Autodesk Fusion 360 part; units mm, degrees
(part 3 of 5)
  spline S32 degree 5 poles (96.0186, 106.2511) (96.0621, 106.2993) (96.1478, 106.3966) (96.2726, 106.5457) (96.4317, 106.7503) (96.6205, 107.0141) (96.8023, 107.2836) (96.9796, 107.5565) (97.1546, 107.8314) (97.328, 108.1075) (97.4996, 108.3849) (97.6689, 108.664) (97.8352, 108.9454) (97.9978, 109.2294) (98.1569, 109.5161) (98.3127, 109.8051) (98.4657, 110.0962) (98.6162, 110.389) (98.7647, 110.6831) (98.9112, 110.9786) (99.0558, 111.2754) (99.1982, 111.5737) (99.3383, 111.8734) (99.4762, 112.1746) (99.6118, 112.4773) (99.7453, 112.7815) (99.8767, 113.0869) (100.0061, 113.3936) (100.1336, 113.7015) (100.2592, 114.0106) (100.383, 114.3207) (100.5049, 114.6321) (100.6249, 114.9445) (100.7431, 115.2581) (100.8594, 115.5727) (100.974, 115.8885) (101.0867, 116.2052) (101.1977, 116.523) (101.3069, 116.8418) (101.4144, 117.1615) (101.5203, 117.4822) (101.6244, 117.8038) (101.7269, 118.1263) (101.8276, 118.4498) (101.9268, 118.7742) (102.0242, 119.0994) (102.1201, 119.4255) (102.2143, 119.7524) (102.307, 120.0802) (102.398, 120.4088) (102.4875, 120.7382) (102.5754, 121.0684) (102.6617, 121.3994) (102.7465, 121.7312) (102.8297, 122.0637) (102.9114, 122.397) (102.9916, 122.731) (103.0703, 123.0657) (103.1474, 123.4011) (103.2231, 123.7373) (103.2972, 124.0741) (103.3699, 124.4117) (103.4411, 124.7499) (103.5108, 125.0888) (103.5791, 125.4283) (103.6459, 125.7685) (103.7112, 126.1093) (103.7751, 126.4508) (103.8376, 126.7928) (103.8986, 127.1355) (103.9582, 127.4788) (104.0048, 127.7539) (104.039, 127.9605) (104.0616, 128.0984) (104.0728, 128.1673) knots 0 0 0 0 0 0 0.01428571 0.02857143 0.04285714 0.05714286 0.07142857 0.08571429 0.1 0.11428571 0.12857143 0.14285714 0.15714286 0.17142857 0.18571429 0.2 0.21428571 0.22857143 0.24285714 0.25714286 0.27142857 0.28571429 0.3 0.31428571 0.32857143 0.34285714 0.35714286 0.37142857 0.38571429 0.4 0.41428571 0.42857143 0.44285714 0.45714286 0.47142857 0.48571429 0.5 0.51428571 0.52857143 0.54285714 0.55714286 0.57142857 0.58571429 0.6 0.61428571 0.62857143 0.64285714 0.65714286 0.67142857 0.68571429 0.7 0.71428571 0.72857143 0.74285714 0.75714286 0.77142857 0.78571429 0.8 0.81428571 0.82857143 0.84285714 0.85714286 0.87142857 0.88571429 0.9 0.91428571 0.92857143 0.94285714 0.95714286 0.97142857 0.98571429 1 1 1 1 1 1
  arc A66 (104.0728, 128.1673) -> (96.8641, 133.6987) centre (0, 0) ccw
  spline S33 degree 5 poles (96.8641, 133.6987) (96.8004, 133.6701) (96.6731, 133.6126) (96.4824, 133.526) (96.2287, 133.4099) (95.9125, 133.2634) (95.5973, 133.1158) (95.2831, 132.9669) (94.9698, 132.8168) (94.6575, 132.6655) (94.3462, 132.5129) (94.0359, 132.3591) (93.7266, 132.2041) (93.4184, 132.0478) (93.1111, 131.8902) (92.805, 131.7314) (92.4998, 131.5713) (92.1958, 131.41) (91.8928, 131.2474) (91.5909, 131.0835) (91.2902, 130.9183) (90.9905, 130.7518) (90.692, 130.5841) (90.3946, 130.415) (90.0984, 130.2447) (89.8034, 130.073) (89.5096, 129.9) (89.2169, 129.7257) (88.9255, 129.55) (88.6354, 129.373) (88.3464, 129.1947) (88.0588, 129.015) (87.7724, 128.8339) (87.4874, 128.6515) (87.2037, 128.4677) (86.9213, 128.2824) (86.6403, 128.0958) (86.3607, 127.9078) (86.0825, 127.7184) (85.8057, 127.5275) (85.5303, 127.3352) (85.2565, 127.1414) (84.9842, 126.9461) (84.7135, 126.7492) (84.4443, 126.5509) (84.1768, 126.3511) (83.9108, 126.1497) (83.6464, 125.9469) (83.3836, 125.7425) (83.1225, 125.5365) (82.8633, 125.3289) (82.606, 125.1196) (82.3507, 124.9084) (82.0975, 124.6954) (81.8463, 124.4807) (81.597, 124.2643) (81.3495, 124.0463) (81.1038, 123.8267) (80.86, 123.6055) (80.6184, 123.3824) (80.3795, 123.1571) (80.1438, 122.9293) (79.9116, 122.6986) (79.6828, 122.4652) (79.457, 122.2295) (79.2335, 121.9919) (79.0117, 121.7529) (78.7915, 121.5128) (78.5737, 121.2708) (78.3604, 121.0256) (78.1545, 120.7749) (77.998, 120.5683) (77.8863, 120.4091) (77.8145, 120.3011) (77.7792, 120.2466) knots -1 -1 -1 -1 -1 -1 -0.98571429 -0.97142857 -0.95714286 -0.94285714 -0.92857143 -0.91428571 -0.9 -0.88571429 -0.87142857 -0.85714286 -0.84285714 -0.82857143 -0.81428571 -0.8 -0.78571429 -0.77142857 -0.75714286 -0.74285714 -0.72857143 -0.71428571 -0.7 -0.68571429 -0.67142857 -0.65714286 -0.64285714 -0.62857143 -0.61428571 -0.6 -0.58571429 -0.57142857 -0.55714286 -0.54285714 -0.52857143 -0.51428571 -0.5 -0.48571429 -0.47142857 -0.45714286 -0.44285714 -0.42857143 -0.41428571 -0.4 -0.38571429 -0.37142857 -0.35714286 -0.34285714 -0.32857143 -0.31428571 -0.3 -0.28571429 -0.27142857 -0.25714286 -0.24285714 -0.22857143 -0.21428571 -0.2 -0.18571429 -0.17142857 -0.15714286 -0.14285714 -0.12857143 -0.11428571 -0.1 -0.08571429 -0.07142857 -0.05714286 -0.04285714 -0.02857143 -0.01428571 0 0 0 0 0 0
  line L33 (77.7792, 120.2466) -> (75.8689, 117.2932)
  arc A67 (73.1275, 116.6848) -> (75.8689, 117.2932) centre (74.1896, 118.3795) ccw
  arc A68 (73.1275, 116.6848) -> (64.4882, 121.6727) centre (0, 0) ccw
  arc A69 (63.6445, 124.351) -> (64.4882, 121.6727) centre (65.4248, 123.4398) ccw
  line L34 (63.6445, 124.351) -> (65.247, 127.4821)
  spline S34 degree 5 poles (65.247, 127.4821) (65.2766, 127.5399) (65.3342, 127.6561) (65.4162, 127.8324) (65.5168, 128.0712) (65.631, 128.3749) (65.7368, 128.6822) (65.8374, 128.9918) (65.9353, 129.3026) (66.0313, 129.6142) (66.1253, 129.9265) (66.2166, 130.2399) (66.3044, 130.5548) (66.388, 130.8712) (66.4674, 131.1893) (66.5431, 131.5088) (66.6155, 131.8296) (66.6852, 132.1513) (66.7525, 132.4739) (66.8175, 132.7972) (66.8803, 133.1213) (66.9407, 133.4463) (66.9985, 133.772) (67.0537, 134.0987) (67.1064, 134.4262) (67.1565, 134.7545) (67.2044, 135.0836) (67.25, 135.4133) (67.2935, 135.7437) (67.3349, 136.0747) (67.3741, 136.4064) (67.4113, 136.7386) (67.4464, 137.0715) (67.4794, 137.405) (67.5103, 137.739) (67.5392, 138.0736) (67.5661, 138.4088) (67.5911, 138.7445) (67.6141, 139.0806) (67.6352, 139.4173) (67.6544, 139.7544) (67.6718, 140.0921) (67.6872, 140.4301) (67.7009, 140.7687) (67.7127, 141.1076) (67.7227, 141.447) (67.7309, 141.7868) (67.7373, 142.127) (67.7419, 142.4676) (67.7448, 142.8085) (67.746, 143.1499) (67.7454, 143.4916) (67.7431, 143.8336) (67.7392, 144.176) (67.7335, 144.5188) (67.7262, 144.8618) (67.7171, 145.2052) (67.7065, 145.5489) (67.6942, 145.8929) (67.6803, 146.2371) (67.6647, 146.5817) (67.6475, 146.9266) (67.6288, 147.2717) (67.6084, 147.6171) (67.5865, 147.9627) (67.5629, 148.3086) (67.5378, 148.6547) (67.5112, 149.001) (67.483, 149.3476) (67.4533, 149.6944) (67.422, 150.0414) (67.3957, 150.3192) (67.3754, 150.5276) (67.3615, 150.6666) (67.3545, 150.7362) knots 0 0 0 0 0 0 0.01428571 0.02857143 0.04285714 0.05714286 0.07142857 0.08571429 0.1 0.11428571 0.12857143 0.14285714 0.15714286 0.17142857 0.18571429 0.2 0.21428571 0.22857143 0.24285714 0.25714286 0.27142857 0.28571429 0.3 0.31428571 0.32857143 0.34285714 0.35714286 0.37142857 0.38571429 0.4 0.41428571 0.42857143 0.44285714 0.45714286 0.47142857 0.48571429 0.5 0.51428571 0.52857143 0.54285714 0.55714286 0.57142857 0.58571429 0.6 0.61428571 0.62857143 0.64285714 0.65714286 0.67142857 0.68571429 0.7 0.71428571 0.72857143 0.74285714 0.75714286 0.77142857 0.78571429 0.8 0.81428571 0.82857143 0.84285714 0.85714286 0.87142857 0.88571429 0.9 0.91428571 0.92857143 0.94285714 0.95714286 0.97142857 0.98571429 1 1 1 1 1 1
  arc A70 (67.3545, 150.7362) -> (58.9598, 154.2133) centre (0, 0) ccw
  spline S35 degree 5 poles (58.9598, 154.2133) (58.9056, 154.1692) (58.7975, 154.0807) (58.6357, 153.9477) (58.4208, 153.7698) (58.1533, 153.5466) (57.887, 153.3224) (57.622, 153.0973) (57.3583, 152.8712) (57.0958, 152.6442) (56.8346, 152.4163) (56.5747, 152.1874) (56.316, 151.9576) (56.0587, 151.7268) (55.8028, 151.4951) (55.5481, 151.2625) (55.2948, 151.0289) (55.0429, 150.7943) (54.7923, 150.5588) (54.5432, 150.3224) (54.2954, 150.085) (54.049, 149.8467) (53.8041, 149.6074) (53.5606, 149.3671) (53.3186, 149.1259) (53.0781, 148.8837) (52.839, 148.6405) (52.6015, 148.3964) (52.3655, 148.1513) (52.131, 147.9053) (51.8981, 147.6582) (51.6667, 147.4102) (51.437, 147.1612) (51.2089, 146.9112) (50.9824, 146.6602) (50.7576, 146.4082) (50.5345, 146.1552) (50.313, 145.9012) (50.0933, 145.6463) (49.8754, 145.3902) (49.6592, 145.1332) (49.4448, 144.8751) (49.2324, 144.616) (49.0218, 144.3558) (48.8132, 144.0946) (48.6064, 143.8323) (48.4016, 143.569) (48.1987, 143.3046) (47.9978, 143.0392) (47.799, 142.7727) (47.6023, 142.505) (47.408, 142.2362) (47.216, 141.9662) (47.0265, 141.695) (46.8395, 141.4225) (46.6547, 141.149) (46.472, 140.8743) (46.2915, 140.5987) (46.1133, 140.3219) (45.9377, 140.0439) (45.7653, 139.7644) (45.5965, 139.4833) (45.4319, 139.2004) (45.2713, 138.9158) (45.1143, 138.6296) (44.9599, 138.3422) (44.8074, 138.054) (44.6569, 137.7651) (44.5092, 137.475) (44.3666, 137.1829) (44.2326, 136.8874) (44.135, 136.6474) (44.0682, 136.4648) (44.0268, 136.3418) (44.0069, 136.2801) knots -1 -1 -1 -1 -1 -1 -0.98571429 -0.97142857 -0.95714286 -0.94285714 -0.92857143 -0.91428571 -0.9 -0.88571429 -0.87142857 -0.85714286 -0.84285714 -0.82857143 -0.81428571 -0.8 -0.78571429 -0.77142857 -0.75714286 -0.74285714 -0.72857143 -0.71428571 -0.7 -0.68571429 -0.67142857 -0.65714286 -0.64285714 -0.62857143 -0.61428571 -0.6 -0.58571429 -0.57142857 -0.55714286 -0.54285714 -0.52857143 -0.51428571 -0.5 -0.48571429 -0.47142857 -0.45714286 -0.44285714 -0.42857143 -0.41428571 -0.4 -0.38571429 -0.37142857 -0.35714286 -0.34285714 -0.32857143 -0.31428571 -0.3 -0.28571429 -0.27142857 -0.25714286 -0.24285714 -0.22857143 -0.21428571 -0.2 -0.18571429 -0.17142857 -0.15714286 -0.14285714 -0.12857143 -0.11428571 -0.1 -0.08571429 -0.07142857 -0.05714286 -0.04285714 -0.02857143 -0.01428571 0 0 0 0 0 0
  line L35 (44.0069, 136.2801) -> (42.926, 132.9329)
  arc A71 (40.4355, 131.6356) -> (42.926, 132.9329) centre (41.0228, 133.5475) ccw
  arc A72 (40.4355, 131.6356) -> (30.7996, 134.2176) centre (0, 0) ccw
  arc A73 (29.2914, 136.5863) -> (30.7996, 134.2176) centre (31.247, 136.1669) ccw
  line L36 (29.2914, 136.5863) -> (30.029, 140.0254)
  spline S36 degree 5 poles (30.029, 140.0254) (30.0426, 140.0889) (30.0682, 140.2161) (30.1017, 140.4076) (30.1371, 140.6643) (30.1688, 140.9872) (30.1914, 141.3114) (30.2085, 141.6365) (30.2226, 141.962) (30.2347, 142.2878) (30.2447, 142.6139) (30.2518, 142.9402) (30.255, 143.267) (30.2539, 143.5944) (30.2483, 143.9222) (30.2387, 144.2504) (30.2257, 144.579) (30.2097, 144.9078) (30.1912, 145.2368) (30.1703, 145.5659) (30.1471, 145.8952) (30.1213, 146.2247) (30.0928, 146.5543) (30.0616, 146.8842) (30.0277, 147.2141) (29.9912, 147.5442) (29.9523, 147.8745) (29.911, 148.2048) (29.8675, 148.5352) (29.8217, 148.8657) (29.7739, 149.1962) (29.7238, 149.5267) (29.6715, 149.8573) (29.6171, 150.188) (29.5605, 150.5186) (29.5018, 150.8493) (29.441, 151.18) (29.3782, 151.5107) (29.3135, 151.8414) (29.2467, 152.172) (29.178, 152.5027) (29.1074, 152.8333) (29.0349, 153.1638) (28.9604, 153.4944) (28.8841, 153.8248) (28.8059, 154.1552) (28.7259, 154.4856) (28.644, 154.8158) (28.5603, 155.146) (28.4749, 155.4761) (28.3877, 155.8061) (28.2987, 156.136) (28.208, 156.4658) (28.1155, 156.7955) (28.0213, 157.1251) (27.9254, 157.4546) (27.8279, 157.7839) (27.7286, 158.1132) (27.6277, 158.4422) (27.5252, 158.7712) (27.4209, 159.1) (27.3151, 159.4286) (27.2077, 159.7571) (27.0986, 160.0855) (26.9879, 160.4136) (26.8757, 160.7417) (26.7619, 161.0695) (26.6465, 161.3971) (26.5296, 161.7246) (26.4111, 162.0519) (26.2911, 162.379) (26.1938, 162.6405) (26.1202, 162.8366) (26.0708, 162.9672) (26.046, 163.0326) knots 0 0 0 0 0 0 0.01428571 0.02857143 0.04285714 0.05714286 0.07142857 0.08571429 0.1 0.11428571 0.12857143 0.14285714 0.15714286 0.17142857 0.18571429 0.2 0.21428571 0.22857143 0.24285714 0.25714286 0.27142857 0.28571429 0.3 0.31428571 0.32857143 0.34285714 0.35714286 0.37142857 0.38571429 0.4 0.41428571 0.42857143 0.44285714 0.45714286 0.47142857 0.48571429 0.5 0.51428571 0.52857143 0.54285714 0.55714286 0.57142857 0.58571429 0.6 0.61428571 0.62857143 0.64285714 0.65714286 0.67142857 0.68571429 0.7 0.71428571 0.72857143 0.74285714 0.75714286 0.77142857 0.78571429 0.8 0.81428571 0.82857143 0.84285714 0.85714286 0.87142857 0.88571429 0.9 0.91428571 0.92857143 0.94285714 0.95714286 0.97142857 0.98571429 1 1 1 1 1 1
  arc A74 (26.046, 163.0326) -> (17.0374, 164.2186) centre (0, 0) ccw
  spline S37 degree 5 poles (17.0374, 164.2186) (16.9966, 164.1619) (16.915, 164.0484) (16.7932, 163.8781) (16.6316, 163.6507) (16.431, 163.3658) (16.2318, 163.0803) (16.0341, 162.7943) (15.8379, 162.5077) (15.6431, 162.2205) (15.4498, 161.9327) (15.2579, 161.6443) (15.0676, 161.3554) (14.8788, 161.0659) (14.6915, 160.7758) (14.5057, 160.4852) (14.3215, 160.194) (14.1389, 159.9023) (13.9578, 159.61) (13.7783, 159.3171) (13.6005, 159.0237) (13.4242, 158.7297) (13.2495, 158.4351) (13.0765, 158.1401) (12.9052, 157.8444) (12.7355, 157.5482) (12.5676, 157.2515) (12.4013, 156.9542) (12.2368, 156.6564) (12.0739, 156.358) (11.9129, 156.0591) (11.7536, 155.7597) (11.5962, 155.4597) (11.4406, 155.1592) (11.2868, 154.8581) (11.1349, 154.5565) (10.9848, 154.2544) (10.8367, 153.9518) (10.6904, 153.6486) (10.5461, 153.3449) (10.4039, 153.0407) (10.2636, 152.7359) (10.1254, 152.4306) (9.9894, 152.1248) (9.8555, 151.8185) (9.7237, 151.5116) (9.594, 151.2043) (9.4664, 150.8964) (9.3411, 150.588) (9.218, 150.2791) (9.0973, 149.9697) (8.9791, 149.6597) (8.8636, 149.3492) (8.7508, 149.0382) (8.6406, 148.7266) (8.5329, 148.4145) (8.4276, 148.102) (8.3246, 147.789) (8.224, 147.4755) (8.1264, 147.1615) (8.0321, 146.847) (7.9419, 146.5318) (7.8561, 146.2159) (7.7747, 145.8994) (7.6971, 145.5823) (7.6223, 145.2648) (7.5497, 144.947) (7.479, 144.6289) (7.4114, 144.3105) (7.3493, 143.9914) (7.2964, 143.6714) (7.2641, 143.4142) (7.247, 143.2205) (7.2388, 143.0911) (7.2355, 143.0263) knots -1 -1 -1 -1 -1 -1 -0.98571429 -0.97142857 -0.95714286 -0.94285714 -0.92857143 -0.91428571 -0.9 -0.88571429 -0.87142857 -0.85714286 -0.84285714 -0.82857143 -0.81428571 -0.8 -0.78571429 -0.77142857 -0.75714286 -0.74285714 -0.72857143 -0.71428571 -0.7 -0.68571429 -0.67142857 -0.65714286 -0.64285714 -0.62857143 -0.61428571 -0.6 -0.58571429 -0.57142857 -0.55714286 -0.54285714 -0.52857143 -0.51428571 -0.5 -0.48571429 -0.47142857 -0.45714286 -0.44285714 -0.42857143 -0.41428571 -0.4 -0.38571429 -0.37142857 -0.35714286 -0.34285714 -0.32857143 -0.31428571 -0.3 -0.28571429 -0.27142857 -0.25714286 -0.24285714 -0.22857143 -0.21428571 -0.2 -0.18571429 -0.17142857 -0.15714286 -0.14285714 -0.12857143 -0.11428571 -0.1 -0.08571429 -0.07142857 -0.05714286 -0.04285714 -0.02857143 -0.01428571 0 0 0 0 0 0
  line L37 (7.2355, 143.0263) -> (7.0578, 139.5134)
  arc A75 (4.9879, 137.6157) -> (7.0578, 139.5134) centre (5.0603, 139.6144) ccw
  arc A76 (4.9879, 137.6157) -> (-4.9879, 137.6157) centre (0, 0) ccw
  arc A77 (-7.0578, 139.5134) -> (-4.9879, 137.6157) centre (-5.0603, 139.6144) ccw
  line L38 (-7.0578, 139.5134) -> (-7.2355, 143.0263)
  spline S38 degree 5 poles (-7.2355, 143.0263) (-7.2388, 143.0911) (-7.247, 143.2205) (-7.2641, 143.4142) (-7.2964, 143.6714) (-7.3493, 143.9914) (-7.4114, 144.3105) (-7.479, 144.6289) (-7.5497, 144.947) (-7.6223, 145.2648) (-7.6971, 145.5823) (-7.7747, 145.8994) (-7.8561, 146.2159) (-7.9419, 146.5318) (-8.0321, 146.847) (-8.1264, 147.1615) (-8.224, 147.4755) (-8.3246, 147.789) (-8.4276, 148.102) (-8.5329, 148.4145) (-8.6406, 148.7266) (-8.7508, 149.0382) (-8.8636, 149.3492) (-8.9791, 149.6597) (-9.0973, 149.9697) (-9.218, 150.2791) (-9.3411, 150.588) (-9.4664, 150.8964) (-9.594, 151.2043) (-9.7237, 151.5116) (-9.8555, 151.8185) (-9.9894, 152.1248) (-10.1254, 152.4306) (-10.2636, 152.7359) (-10.4039, 153.0407) (-10.5461, 153.3449) (-10.6904, 153.6486) (-10.8367, 153.9518) (-10.9848, 154.2544) (-11.1349, 154.5565) (-11.2868, 154.8581) (-11.4406, 155.1592) (-11.5962, 155.4597) (-11.7536, 155.7597) (-11.9129, 156.0591) (-12.0739, 156.358) (-12.2368, 156.6564) (-12.4013, 156.9542) (-12.5676, 157.2515) (-12.7355, 157.5482) (-12.9052, 157.8444) (-13.0765, 158.1401) (-13.2495, 158.4351) (-13.4242, 158.7297) (-13.6005, 159.0237) (-13.7783, 159.3171) (-13.9578, 159.61) (-14.1389, 159.9023) (-14.3215, 160.194) (-14.5057, 160.4852) (-14.6915, 160.7758) (-14.8788, 161.0659) (-15.0676, 161.3554) (-15.2579, 161.6443) (-15.4498, 161.9327) (-15.6431, 162.2205) (-15.8379, 162.5077) (-16.0341, 162.7943) (-16.2318, 163.0803) (-16.431, 163.3658) (-16.6316, 163.6507) (-16.7932, 163.8781) (-16.915, 164.0484) (-16.9966, 164.1619) (-17.0374, 164.2186) knots 0 0 0 0 0 0 0.01428571 0.02857143 0.04285714 0.05714286 0.07142857 0.08571429 0.1 0.11428571 0.12857143 0.14285714 0.15714286 0.17142857 0.18571429 0.2 0.21428571 0.22857143 0.24285714 0.25714286 0.27142857 0.28571429 0.3 0.31428571 0.32857143 0.34285714 0.35714286 0.37142857 0.38571429 0.4 0.41428571 0.42857143 0.44285714 0.45714286 0.47142857 0.48571429 0.5 0.51428571 0.52857143 0.54285714 0.55714286 0.57142857 0.58571429 0.6 0.61428571 0.62857143 0.64285714 0.65714286 0.67142857 0.68571429 0.7 0.71428571 0.72857143 0.74285714 0.75714286 0.77142857 0.78571429 0.8 0.81428571 0.82857143 0.84285714 0.85714286 0.87142857 0.88571429 0.9 0.91428571 0.92857143 0.94285714 0.95714286 0.97142857 0.98571429 1 1 1 1 1 1
  arc A78 (-17.0374, 164.2186) -> (-26.046, 163.0326) centre (0, 0) ccw
  spline S39 degree 5 poles (-26.046, 163.0326) (-26.0708, 162.9672) (-26.1202, 162.8366) (-26.1938, 162.6405) (-26.2911, 162.379) (-26.4111, 162.0519) (-26.5296, 161.7246) (-26.6465, 161.3971) (-26.7619, 161.0695) (-26.8757, 160.7417) (-26.9879, 160.4136) (-27.0986, 160.0855) (-27.2077, 159.7571) (-27.3151, 159.4286) (-27.4209, 159.1) (-27.5252, 158.7712) (-27.6277, 158.4422) (-27.7286, 158.1132) (-27.8279, 157.7839) (-27.9254, 157.4546) (-28.0213, 157.1251) (-28.1155, 156.7955) (-28.208, 156.4658) (-28.2987, 156.136) (-28.3877, 155.8061) (-28.4749, 155.4761) (-28.5603, 155.146) (-28.644, 154.8158) (-28.7259, 154.4856) (-28.8059, 154.1552) (-28.8841, 153.8248) (-28.9604, 153.4944) (-29.0349, 153.1638) (-29.1074, 152.8333) (-29.178, 152.5027) (-29.2467, 152.172) (-29.3135, 151.8414) (-29.3782, 151.5107) (-29.441, 151.18) (-29.5018, 150.8493) (-29.5605, 150.5186) (-29.6171, 150.188) (-29.6715, 149.8573) (-29.7238, 149.5267) (-29.7739, 149.1962) (-29.8217, 148.8657) (-29.8675, 148.5352) (-29.911, 148.2048) (-29.9523, 147.8745) (-29.9912, 147.5442) (-30.0277, 147.2141) (-30.0616, 146.8842) (-30.0928, 146.5543) (-30.1213, 146.2247) (-30.1471, 145.8952) (-30.1703, 145.5659) (-30.1912, 145.2368) (-30.2097, 144.9078) (-30.2257, 144.579) (-30.2387, 144.2504) (-30.2483, 143.9222) (-30.2539, 143.5944) (-30.255, 143.267) (-30.2518, 142.9402) (-30.2447, 142.6139) (-30.2347, 142.2878) (-30.2226, 141.962) (-30.2085, 141.6365) (-30.1914, 141.3114) (-30.1688, 140.9872) (-30.1371, 140.6643) (-30.1017, 140.4076) (-30.0682, 140.2161) (-30.0426, 140.0889) (-30.029, 140.0254) knots -1 -1 -1 -1 -1 -1 -0.98571429 -0.97142857 -0.95714286 -0.94285714 -0.92857143 -0.91428571 -0.9 -0.88571429 -0.87142857 -0.85714286 -0.84285714 -0.82857143 -0.81428571 -0.8 -0.78571429 -0.77142857 -0.75714286 -0.74285714 -0.72857143 -0.71428571 -0.7 -0.68571429 -0.67142857 -0.65714286 -0.64285714 -0.62857143 -0.61428571 -0.6 -0.58571429 -0.57142857 -0.55714286 -0.54285714 -0.52857143 -0.51428571 -0.5 -0.48571429 -0.47142857 -0.45714286 -0.44285714 -0.42857143 -0.41428571 -0.4 -0.38571429 -0.37142857 -0.35714286 -0.34285714 -0.32857143 -0.31428571 -0.3 -0.28571429 -0.27142857 -0.25714286 -0.24285714 -0.22857143 -0.21428571 -0.2 -0.18571429 -0.17142857 -0.15714286 -0.14285714 -0.12857143 -0.11428571 -0.1 -0.08571429 -0.07142857 -0.05714286 -0.04285714 -0.02857143 -0.01428571 0 0 0 0 0 0
  line L39 (-30.029, 140.0254) -> (-29.2914, 136.5863)
  arc A79 (-30.7996, 134.2176) -> (-29.2914, 136.5863) centre (-31.247, 136.1669) ccw
  arc A80 (-30.7996, 134.2176) -> (-40.4355, 131.6356) centre (0, 0) ccw
  arc A81 (-42.926, 132.9329) -> (-40.4355, 131.6356) centre (-41.0228, 133.5475) ccw
  line L40 (-42.926, 132.9329) -> (-44.0069, 136.2801)
  spline S40 degree 5 poles (-44.0069, 136.2801) (-44.0268, 136.3418) (-44.0682, 136.4648) (-44.135, 136.6474) (-44.2326, 136.8874) (-44.3666, 137.1829) (-44.5092, 137.475) (-44.6569, 137.7651) (-44.8074, 138.054) (-44.9599, 138.3422) (-45.1143, 138.6296) (-45.2713, 138.9158) (-45.4319, 139.2004) (-45.5965, 139.4833) (-45.7653, 139.7644) (-45.9377, 140.0439) (-46.1133, 140.3219) (-46.2915, 140.5987) (-46.472, 140.8743) (-46.6547, 141.149) (-46.8395, 141.4225) (-47.0265, 141.695) (-47.216, 141.9662) (-47.408, 142.2362) (-47.6023, 142.505) (-47.799, 142.7727) (-47.9978, 143.0392) (-48.1987, 143.3046) (-48.4016, 143.569) (-48.6064, 143.8323) (-48.8132, 144.0946) (-49.0218, 144.3558) (-49.2324, 144.616) (-49.4448, 144.8751) (-49.6592, 145.1332) (-49.8754, 145.3902) (-50.0933, 145.6463) (-50.313, 145.9012) (-50.5345, 146.1552) (-50.7576, 146.4082) (-50.9824, 146.6602) (-51.2089, 146.9112) (-51.437, 147.1612) (-51.6667, 147.4102) (-51.8981, 147.6582) (-52.131, 147.9053) (-52.3655, 148.1513) (-52.6015, 148.3964) (-52.839, 148.6405) (-53.0781, 148.8837) (-53.3186, 149.1259) (-53.5606, 149.3671) (-53.8041, 149.6074) (-54.049, 149.8467) (-54.2954, 150.085) (-54.5432, 150.3224) (-54.7923, 150.5588) (-55.0429, 150.7943) (-55.2948, 151.0289) (-55.5481, 151.2625) (-55.8028, 151.4951) (-56.0587, 151.7268) (-56.316, 151.9576) (-56.5747, 152.1874) (-56.8346, 152.4163) (-57.0958, 152.6442) (-57.3583, 152.8712) (-57.622, 153.0973) (-57.887, 153.3224) (-58.1533, 153.5466) (-58.4208, 153.7698) (-58.6357, 153.9477) (-58.7975, 154.0807) (-58.9056, 154.1692) (-58.9598, 154.2133) knots 0 0 0 0 0 0 0.01428571 0.02857143 0.04285714 0.05714286 0.07142857 0.08571429 0.1 0.11428571 0.12857143 0.14285714 0.15714286 0.17142857 0.18571429 0.2 0.21428571 0.22857143 0.24285714 0.25714286 0.27142857 0.28571429 0.3 0.31428571 0.32857143 0.34285714 0.35714286 0.37142857 0.38571429 0.4 0.41428571 0.42857143 0.44285714 0.45714286 0.47142857 0.48571429 0.5 0.51428571 0.52857143 0.54285714 0.55714286 0.57142857 0.58571429 0.6 0.61428571 0.62857143 0.64285714 0.65714286 0.67142857 0.68571429 0.7 0.71428571 0.72857143 0.74285714 0.75714286 0.77142857 0.78571429 0.8 0.81428571 0.82857143 0.84285714 0.85714286 0.87142857 0.88571429 0.9 0.91428571 0.92857143 0.94285714 0.95714286 0.97142857 0.98571429 1 1 1 1 1 1
  arc A82 (-58.9598, 154.2133) -> (-67.3545, 150.7362) centre (0, 0) ccw
  spline S41 degree 5 poles (-67.3545, 150.7362) (-67.3615, 150.6666) (-67.3754, 150.5276) (-67.3957, 150.3192) (-67.422, 150.0414) (-67.4533, 149.6944) (-67.483, 149.3476) (-67.5112, 149.001) (-67.5378, 148.6547) (-67.5629, 148.3086) (-67.5865, 147.9627) (-67.6084, 147.6171) (-67.6288, 147.2717) (-67.6475, 146.9266) (-67.6647, 146.5817) (-67.6803, 146.2371) (-67.6942, 145.8929) (-67.7065, 145.5489) (-67.7171, 145.2052) (-67.7262, 144.8618) (-67.7335, 144.5188) (-67.7392, 144.176) (-67.7431, 143.8336) (-67.7454, 143.4916) (-67.746, 143.1499) (-67.7448, 142.8085) (-67.7419, 142.4676) (-67.7373, 142.127) (-67.7309, 141.7868) (-67.7227, 141.447) (-67.7127, 141.1076) (-67.7009, 140.7687) (-67.6872, 140.4301) (-67.6718, 140.0921) (-67.6544, 139.7544) (-67.6352, 139.4173) (-67.6141, 139.0806) (-67.5911, 138.7445) (-67.5661, 138.4088) (-67.5392, 138.0736) (-67.5103, 137.739) (-67.4794, 137.405) (-67.4464, 137.0715) (-67.4113, 136.7386) (-67.3741, 136.4064) (-67.3349, 136.0747) (-67.2935, 135.7437) (-67.25, 135.4133) (-67.2044, 135.0836) (-67.1565, 134.7545) (-67.1064, 134.4262) (-67.0537, 134.0987) (-66.9985, 133.772) (-66.9407, 133.4463) (-66.8803, 133.1213) (-66.8175, 132.7972) (-66.7525, 132.4739) (-66.6852, 132.1513) (-66.6155, 131.8296) (-66.5431, 131.5088) (-66.4674, 131.1893) (-66.388, 130.8712) (-66.3044, 130.5548) (-66.2166, 130.2399) (-66.1253, 129.9265) (-66.0313, 129.6142) (-65.9353, 129.3026) (-65.8374, 128.9918) (-65.7368, 128.6822) (-65.631, 128.3749) (-65.5168, 128.0712) (-65.4162, 127.8324) (-65.3342, 127.6561) (-65.2766, 127.5399) (-65.247, 127.4821) knots -1 -1 -1 -1 -1 -1 -0.98571429 -0.97142857 -0.95714286 -0.94285714 -0.92857143 -0.91428571 -0.9 -0.88571429 -0.87142857 -0.85714286 -0.84285714 -0.82857143 -0.81428571 -0.8 -0.78571429 -0.77142857 -0.75714286 -0.74285714 -0.72857143 -0.71428571 -0.7 -0.68571429 -0.67142857 -0.65714286 -0.64285714 -0.62857143 -0.61428571 -0.6 -0.58571429 -0.57142857 -0.55714286 -0.54285714 -0.52857143 -0.51428571 -0.5 -0.48571429 -0.47142857 -0.45714286 -0.44285714 -0.42857143 -0.41428571 -0.4 -0.38571429 -0.37142857 -0.35714286 -0.34285714 -0.32857143 -0.31428571 -0.3 -0.28571429 -0.27142857 -0.25714286 -0.24285714 -0.22857143 -0.21428571 -0.2 -0.18571429 -0.17142857 -0.15714286 -0.14285714 -0.12857143 -0.11428571 -0.1 -0.08571429 -0.07142857 -0.05714286 -0.04285714 -0.02857143 -0.01428571 0 0 0 0 0 0
  line L41 (-65.247, 127.4821) -> (-63.6445, 124.351)
  arc A83 (-64.4882, 121.6727) -> (-63.6445, 124.351) centre (-65.4248, 123.4398) ccw
  arc A84 (-64.4882, 121.6727) -> (-73.1275, 116.6848) centre (0, 0) ccw
  arc A85 (-75.8689, 117.2932) -> (-73.1275, 116.6848) centre (-74.1896, 118.3795) ccw
  line L42 (-75.8689, 117.2932) -> (-77.7792, 120.2466)
  spline S42 degree 5 poles (-77.7792, 120.2466) (-77.8145, 120.3011) (-77.8863, 120.4091) (-77.998, 120.5683) (-78.1545, 120.7749) (-78.3604, 121.0256) (-78.5737, 121.2708) (-78.7915, 121.5128) (-79.0117, 121.7529) (-79.2335, 121.9919) (-79.457, 122.2295) (-79.6828, 122.4652) (-79.9116, 122.6986) (-80.1438, 122.9293) (-80.3795, 123.1571) (-80.6184, 123.3824) (-80.86, 123.6055) (-81.1038, 123.8267) (-81.3495, 124.0463) (-81.597, 124.2643) (-81.8463, 124.4807) (-82.0975, 124.6954) (-82.3507, 124.9084) (-82.606, 125.1196) (-82.8633, 125.3289) (-83.1225, 125.5365) (-83.3836, 125.7425) (-83.6464, 125.9469) (-83.9108, 126.1497) (-84.1768, 126.3511) (-84.4443, 126.5509) (-84.7135, 126.7492) (-84.9842, 126.9461) (-85.2565, 127.1414) (-85.5303, 127.3352) (-85.8057, 127.5275) (-86.0825, 127.7184) (-86.3607, 127.9078) (-86.6403, 128.0958) (-86.9213, 128.2824) (-87.2037, 128.4677) (-87.4874, 128.6515) (-87.7724, 128.8339) (-88.0588, 129.015) (-88.3464, 129.1947) (-88.6354, 129.373) (-88.9255, 129.55) (-89.2169, 129.7257) (-89.5096, 129.9) (-89.8034, 130.073) (-90.0984, 130.2447) (-90.3946, 130.415) (-90.692, 130.5841) (-90.9905, 130.7518) (-91.2902, 130.9183) (-91.5909, 131.0835) (-91.8928, 131.2474) (-92.1958, 131.41) (-92.4998, 131.5713) (-92.805, 131.7314) (-93.1111, 131.8902) (-93.4184, 132.0478) (-93.7266, 132.2041) (-94.0359, 132.3591) (-94.3462, 132.5129) (-94.6575, 132.6655) (-94.9698, 132.8168) (-95.2831, 132.9669) (-95.5973, 133.1158) (-95.9125, 133.2634) (-96.2287, 133.4099) (-96.4824, 133.526) (-96.6731, 133.6126) (-96.8004, 133.6701) (-96.8641, 133.6987) knots 0 0 0 0 0 0 0.01428571 0.02857143 0.04285714 0.05714286 0.07142857 0.08571429 0.1 0.11428571 0.12857143 0.14285714 0.15714286 0.17142857 0.18571429 0.2 0.21428571 0.22857143 0.24285714 0.25714286 0.27142857 0.28571429 0.3 0.31428571 0.32857143 0.34285714 0.35714286 0.37142857 0.38571429 0.4 0.41428571 0.42857143 0.44285714 0.45714286 0.47142857 0.48571429 0.5 0.51428571 0.52857143 0.54285714 0.55714286 0.57142857 0.58571429 0.6 0.61428571 0.62857143 0.64285714 0.65714286 0.67142857 0.68571429 0.7 0.71428571 0.72857143 0.74285714 0.75714286 0.77142857 0.78571429 0.8 0.81428571 0.82857143 0.84285714 0.85714286 0.87142857 0.88571429 0.9 0.91428571 0.92857143 0.94285714 0.95714286 0.97142857 0.98571429 1 1 1 1 1 1
  arc A86 (-96.8641, 133.6987) -> (-104.0728, 128.1673) centre (0, 0) ccw
  spline S43 degree 5 poles (-104.0728, 128.1673) (-104.0616, 128.0984) (-104.039, 127.9605) (-104.0048, 127.7539) (-103.9582, 127.4788) (-103.8986, 127.1355) (-103.8376, 126.7928) (-103.7751, 126.4508) (-103.7112, 126.1093) (-103.6459, 125.7685) (-103.5791, 125.4283) (-103.5108, 125.0888) (-103.4411, 124.7499) (-103.3699, 124.4117) (-103.2972, 124.0741) (-103.2231, 123.7373) (-103.1474, 123.4011) (-103.0703, 123.0657) (-102.9916, 122.731) (-102.9114, 122.397) (-102.8297, 122.0637) (-102.7465, 121.7312) (-102.6617, 121.3994) (-102.5754, 121.0684) (-102.4875, 120.7382) (-102.398, 120.4088) (-102.307, 120.0802) (-102.2143, 119.7524) (-102.1201, 119.4255) (-102.0242, 119.0994) (-101.9268, 118.7742) (-101.8276, 118.4498) (-101.7269, 118.1263) (-101.6244, 117.8038) (-101.5203, 117.4822) (-101.4144, 117.1615) (-101.3069, 116.8418) (-101.1977, 116.523) (-101.0867, 116.2052) (-100.974, 115.8885) (-100.8594, 115.5727) (-100.7431, 115.2581) (-100.6249, 114.9445) (-100.5049, 114.6321) (-100.383, 114.3207) (-100.2592, 114.0106) (-100.1336, 113.7015) (-100.0061, 113.3936) (-99.8767, 113.0869) (-99.7453, 112.7815) (-99.6118, 112.4773) (-99.4762, 112.1746) (-99.3383, 111.8734) (-99.1982, 111.5737) (-99.0558, 111.2754) (-98.9112, 110.9786) (-98.7647, 110.6831) (-98.6162, 110.389) (-98.4657, 110.0962) (-98.3127, 109.8051) (-98.1569, 109.5161) (-97.9978, 109.2294) (-97.8352, 108.9454) (-97.6689, 108.664) (-97.4996, 108.3849) (-97.328, 108.1075) (-97.1546, 107.8314) (-96.9796, 107.5565) (-96.8023, 107.2836) (-96.6205, 107.0141) (-96.4317, 106.7503) (-96.2726, 106.5457) (-96.1478, 106.3966) (-96.0621, 106.2993) (-96.0186, 106.2511) knots -1 -1 -1 -1 -1 -1 -0.98571429 -0.97142857 -0.95714286 -0.94285714 -0.92857143 -0.91428571 -0.9 -0.88571429 -0.87142857 -0.85714286 -0.84285714 -0.82857143 -0.81428571 -0.8 -0.78571429 -0.77142857 -0.75714286 -0.74285714 -0.72857143 -0.71428571 -0.7 -0.68571429 -0.67142857 -0.65714286 -0.64285714 -0.62857143 -0.61428571 -0.6 -0.58571429 -0.57142857 -0.55714286 -0.54285714 -0.52857143 -0.51428571 -0.5 -0.48571429 -0.47142857 -0.45714286 -0.44285714 -0.42857143 -0.41428571 -0.4 -0.38571429 -0.37142857 -0.35714286 -0.34285714 -0.32857143 -0.31428571 -0.3 -0.28571429 -0.27142857 -0.25714286 -0.24285714 -0.22857143 -0.21428571 -0.2 -0.18571429 -0.17142857 -0.15714286 -0.14285714 -0.12857143 -0.11428571 -0.1 -0.08571429 -0.07142857 -0.05714286 -0.04285714 -0.02857143 -0.01428571 0 0 0 0 0 0
  line L43 (-96.0186, 106.2511) -> (-93.6603, 103.6415)
  arc A87 (-93.782, 100.836) -> (-93.6603, 103.6415) centre (-95.1441, 102.3005) ccw
  arc A88 (-93.782, 100.836) -> (-100.836, 93.782) centre (0, 0) ccw
  arc A89 (-103.6415, 93.6603) -> (-100.836, 93.782) centre (-102.3005, 95.1441) ccw
  line L44 (-103.6415, 93.6603) -> (-106.2511, 96.0186)
  spline S44 degree 5 poles (-106.2511, 96.0186) (-106.2993, 96.0621) (-106.3966, 96.1478) (-106.5457, 96.2726) (-106.7503, 96.4317) (-107.0141, 96.6205) (-107.2836, 96.8023) (-107.5565, 96.9796) (-107.8314, 97.1546) (-108.1075, 97.328) (-108.3849, 97.4996) (-108.664, 97.6689) (-108.9454, 97.8352) (-109.2294, 97.9978) (-109.5161, 98.1569) (-109.8051, 98.3127) (-110.0962, 98.4657) (-110.389, 98.6162) (-110.6831, 98.7647) (-110.9786, 98.9112) (-111.2754, 99.0558) (-111.5737, 99.1982) (-111.8734, 99.3383) (-112.1746, 99.4762) (-112.4773, 99.6118) (-112.7815, 99.7453) (-113.0869, 99.8767) (-113.3936, 100.0061) (-113.7015, 100.1336) (-114.0106, 100.2592) (-114.3207, 100.383) (-114.6321, 100.5049) (-114.9445, 100.6249) (-115.2581, 100.7431) (-115.5727, 100.8594) (-115.8885, 100.974) (-116.2052, 101.0867) (-116.523, 101.1977) (-116.8418, 101.3069) (-117.1615, 101.4144) (-117.4822, 101.5203) (-117.8038, 101.6244) (-118.1263, 101.7269) (-118.4498, 101.8276) (-118.7742, 101.9268) (-119.0994, 102.0242) (-119.4255, 102.1201) (-119.7524, 102.2143) (-120.0802, 102.307) (-120.4088, 102.398) (-120.7382, 102.4875) (-121.0684, 102.5754) (-121.3994, 102.6617) (-121.7312, 102.7465) (-122.0637, 102.8297) (-122.397, 102.9114) (-122.731, 102.9916) (-123.0657, 103.0703) (-123.4011, 103.1474) (-123.7373, 103.2231) (-124.0741, 103.2972) (-124.4117, 103.3699) (-124.7499, 103.4411) (-125.0888, 103.5108) (-125.4283, 103.5791) (-125.7685, 103.6459) (-126.1093, 103.7112) (-126.4508, 103.7751) (-126.7928, 103.8376) (-127.1355, 103.8986) (-127.4788, 103.9582) (-127.7539, 104.0048) (-127.9605, 104.039) (-128.0984, 104.0616) (-128.1673, 104.0728) knots 0 0 0 0 0 0 0.01428571 0.02857143 0.04285714 0.05714286 0.07142857 0.08571429 0.1 0.11428571 0.12857143 0.14285714 0.15714286 0.17142857 0.18571429 0.2 0.21428571 0.22857143 0.24285714 0.25714286 0.27142857 0.28571429 0.3 0.31428571 0.32857143 0.34285714 0.35714286 0.37142857 0.38571429 0.4 0.41428571 0.42857143 0.44285714 0.45714286 0.47142857 0.48571429 0.5 0.51428571 0.52857143 0.54285714 0.55714286 0.57142857 0.58571429 0.6 0.61428571 0.62857143 0.64285714 0.65714286 0.67142857 0.68571429 0.7 0.71428571 0.72857143 0.74285714 0.75714286 0.77142857 0.78571429 0.8 0.81428571 0.82857143 0.84285714 0.85714286 0.87142857 0.88571429 0.9 0.91428571 0.92857143 0.94285714 0.95714286 0.97142857 0.98571429 1 1 1 1 1 1
  arc A90 (-128.1673, 104.0728) -> (-133.6987, 96.8641) centre (0, 0) ccw
  spline S45 degree 5 poles (-133.6987, 96.8641) (-133.6701, 96.8004) (-133.6126, 96.6731) (-133.526, 96.4824) (-133.4099, 96.2287) (-133.2634, 95.9125) (-133.1158, 95.5973) (-132.9669, 95.2831) (-132.8168, 94.9698) (-132.6655, 94.6575) (-132.5129, 94.3462) (-132.3591, 94.0359) (-132.2041, 93.7266) (-132.0478, 93.4184) (-131.8902, 93.1111) (-131.7314, 92.805) (-131.5713, 92.4998) (-131.41, 92.1958) (-131.2474, 91.8928) (-131.0835, 91.5909) (-130.9183, 91.2902) (-130.7518, 90.9905) (-130.5841, 90.692) (-130.415, 90.3946) (-130.2447, 90.0984) (-130.073, 89.8034) (-129.9, 89.5096) (-129.7257, 89.2169) (-129.55, 88.9255) (-129.373, 88.6354) (-129.1947, 88.3464) (-129.015, 88.0588) (-128.8339, 87.7724) (-128.6515, 87.4874) (-128.4677, 87.2037) (-128.2824, 86.9213) (-128.0958, 86.6403) (-127.9078, 86.3607) (-127.7184, 86.0825) (-127.5275, 85.8057) (-127.3352, 85.5303) (-127.1414, 85.2565) (-126.9461, 84.9842) (-126.7492, 84.7135) (-126.5509, 84.4443) (-126.3511, 84.1768) (-126.1497, 83.9108) (-125.9469, 83.6464) (-125.7425, 83.3836) (-125.5365, 83.1225) (-125.3289, 82.8633) (-125.1196, 82.606) (-124.9084, 82.3507) (-124.6954, 82.0975) (-124.4807, 81.8463) (-124.2643, 81.597) (-124.0463, 81.3495) (-123.8267, 81.1038) (-123.6055, 80.86) (-123.3824, 80.6184) (-123.1571, 80.3795) (-122.9293, 80.1438) (-122.6986, 79.9116) (-122.4652, 79.6828) (-122.2295, 79.457) (-121.9919, 79.2335) (-121.7529, 79.0117) (-121.5128, 78.7915) (-121.2708, 78.5737) (-121.0256, 78.3604) (-120.7749, 78.1545) (-120.5683, 77.998) (-120.4091, 77.8863) (-120.3011, 77.8145) (-120.2466, 77.7792) knots -1 -1 -1 -1 -1 -1 -0.98571429 -0.97142857 -0.95714286 -0.94285714 -0.92857143 -0.91428571 -0.9 -0.88571429 -0.87142857 -0.85714286 -0.84285714 -0.82857143 -0.81428571 -0.8 -0.78571429 -0.77142857 -0.75714286 -0.74285714 -0.72857143 -0.71428571 -0.7 -0.68571429 -0.67142857 -0.65714286 -0.64285714 -0.62857143 -0.61428571 -0.6 -0.58571429 -0.57142857 -0.55714286 -0.54285714 -0.52857143 -0.51428571 -0.5 -0.48571429 -0.47142857 -0.45714286 -0.44285714 -0.42857143 -0.41428571 -0.4 -0.38571429 -0.37142857 -0.35714286 -0.34285714 -0.32857143 -0.31428571 -0.3 -0.28571429 -0.27142857 -0.25714286 -0.24285714 -0.22857143 -0.21428571 -0.2 -0.18571429 -0.17142857 -0.15714286 -0.14285714 -0.12857143 -0.11428571 -0.1 -0.08571429 -0.07142857 -0.05714286 -0.04285714 -0.02857143 -0.01428571 0 0 0 0 0 0
  line L45 (-120.2466, 77.7792) -> (-117.2932, 75.8689)
  arc A91 (-116.6848, 73.1275) -> (-117.2932, 75.8689) centre (-118.3795, 74.1896) ccw
  arc A92 (-116.6848, 73.1275) -> (-121.6727, 64.4882) centre (0, 0) ccw
  arc A93 (-124.351, 63.6445) -> (-121.6727, 64.4882) centre (-123.4398, 65.4248) ccw
  line L46 (-124.351, 63.6445) -> (-127.4821, 65.247)
  spline S46 degree 5 poles (-127.4821, 65.247) (-127.5399, 65.2766) (-127.6561, 65.3342) (-127.8324, 65.4162) (-128.0712, 65.5168) (-128.3749, 65.631) (-128.6822, 65.7368) (-128.9918, 65.8374) (-129.3026, 65.9353) (-129.6142, 66.0313) (-129.9265, 66.1253) (-130.2399, 66.2166) (-130.5548, 66.3044) (-130.8712, 66.388) (-131.1893, 66.4674) (-131.5088, 66.5431) (-131.8296, 66.6155) (-132.1513, 66.6852) (-132.4739, 66.7525) (-132.7972, 66.8175) (-133.1213, 66.8803) (-133.4463, 66.9407) (-133.772, 66.9985) (-134.0987, 67.0537) (-134.4262, 67.1064) (-134.7545, 67.1565) (-135.0836, 67.2044) (-135.4133, 67.25) (-135.7437, 67.2935) (-136.0747, 67.3349) (-136.4064, 67.3741) (-136.7386, 67.4113) (-137.0715, 67.4464) (-137.405, 67.4794) (-137.739, 67.5103) (-138.0736, 67.5392) (-138.4088, 67.5661) (-138.7445, 67.5911) (-139.0806, 67.6141) (-139.4173, 67.6352) (-139.7544, 67.6544) (-140.0921, 67.6718) (-140.4301, 67.6872) (-140.7687, 67.7009) (-141.1076, 67.7127) (-141.447, 67.7227) (-141.7868, 67.7309) (-142.127, 67.7373) (-142.4676, 67.7419) (-142.8085, 67.7448) (-143.1499, 67.746) (-143.4916, 67.7454) (-143.8336, 67.7431) (-144.176, 67.7392) (-144.5188, 67.7335) (-144.8618, 67.7262) (-145.2052, 67.7171) (-145.5489, 67.7065) (-145.8929, 67.6942) (-146.2371, 67.6803) (-146.5817, 67.6647) (-146.9266, 67.6475) (-147.2717, 67.6288) (-147.6171, 67.6084) (-147.9627, 67.5865) (-148.3086, 67.5629) (-148.6547, 67.5378) (-149.001, 67.5112) (-149.3476, 67.483) (-149.6944, 67.4533) (-150.0414, 67.422) (-150.3192, 67.3957) (-150.5276, 67.3754) (-150.6666, 67.3615) (-150.7362, 67.3545) knots 0 0 0 0 0 0 0.01428571 0.02857143 0.04285714 0.05714286 0.07142857 0.08571429 0.1 0.11428571 0.12857143 0.14285714 0.15714286 0.17142857 0.18571429 0.2 0.21428571 0.22857143 0.24285714 0.25714286 0.27142857 0.28571429 0.3 0.31428571 0.32857143 0.34285714 0.35714286 0.37142857 0.38571429 0.4 0.41428571 0.42857143 0.44285714 0.45714286 0.47142857 0.48571429 0.5 0.51428571 0.52857143 0.54285714 0.55714286 0.57142857 0.58571429 0.6 0.61428571 0.62857143 0.64285714 0.65714286 0.67142857 0.68571429 0.7 0.71428571 0.72857143 0.74285714 0.75714286 0.77142857 0.78571429 0.8 0.81428571 0.82857143 0.84285714 0.85714286 0.87142857 0.88571429 0.9 0.91428571 0.92857143 0.94285714 0.95714286 0.97142857 0.98571429 1 1 1 1 1 1
  arc A94 (-150.7362, 67.3545) -> (-154.2133, 58.9598) centre (0, 0) ccw
  spline S47 degree 5 poles (-154.2133, 58.9598) (-154.1692, 58.9056) (-154.0807, 58.7975) (-153.9477, 58.6357) (-153.7698, 58.4208) (-153.5466, 58.1533) (-153.3224, 57.887) (-153.0973, 57.622) (-152.8712, 57.3583) (-152.6442, 57.0958) (-152.4163, 56.8346) (-152.1874, 56.5747) (-151.9576, 56.316) (-151.7268, 56.0587) (-151.4951, 55.8028) (-151.2625, 55.5481) (-151.0289, 55.2948) (-150.7943, 55.0429) (-150.5588, 54.7923) (-150.3224, 54.5432) (-150.085, 54.2954) (-149.8467, 54.049) (-149.6074, 53.8041) (-149.3671, 53.5606) (-149.1259, 53.3186) (-148.8837, 53.0781) (-148.6405, 52.839) (-148.3964, 52.6015) (-148.1513, 52.3655) (-147.9053, 52.131) (-147.6582, 51.8981) (-147.4102, 51.6667) (-147.1612, 51.437) (-146.9112, 51.2089) (-146.6602, 50.9824) (-146.4082, 50.7576) (-146.1552, 50.5345) (-145.9012, 50.313) (-145.6463, 50.0933) (-145.3902, 49.8754) (-145.1332, 49.6592) (-144.8751, 49.4448) (-144.616, 49.2324) (-144.3558, 49.0218) (-144.0946, 48.8132) (-143.8323, 48.6064) (-143.569, 48.4016) (-143.3046, 48.1987) (-143.0392, 47.9978) (-142.7727, 47.799) (-142.505, 47.6023) (-142.2362, 47.408) (-141.9662, 47.216) (-141.695, 47.0265) (-141.4225, 46.8395) (-141.149, 46.6547) (-140.8743, 46.472) (-140.5987, 46.2915) (-140.3219, 46.1133) (-140.0439, 45.9377) (-139.7644, 45.7653) (-139.4833, 45.5965) (-139.2004, 45.4319) (-138.9158, 45.2713) (-138.6296, 45.1143) (-138.3422, 44.9599) (-138.054, 44.8074) (-137.7651, 44.6569) (-137.475, 44.5092) (-137.1829, 44.3666) (-136.8874, 44.2326) (-136.6474, 44.135) (-136.4648, 44.0682) (-136.3418, 44.0268) (-136.2801, 44.0069) knots -1 -1 -1 -1 -1 -1 -0.98571429 -0.97142857 -0.95714286 -0.94285714 -0.92857143 -0.91428571 -0.9 -0.88571429 -0.87142857 -0.85714286 -0.84285714 -0.82857143 -0.81428571 -0.8 -0.78571429 -0.77142857 -0.75714286 -0.74285714 -0.72857143 -0.71428571 -0.7 -0.68571429 -0.67142857 -0.65714286 -0.64285714 -0.62857143 -0.61428571 -0.6 -0.58571429 -0.57142857 -0.55714286 -0.54285714 -0.52857143 -0.51428571 -0.5 -0.48571429 -0.47142857 -0.45714286 -0.44285714 -0.42857143 -0.41428571 -0.4 -0.38571429 -0.37142857 -0.35714286 -0.34285714 -0.32857143 -0.31428571 -0.3 -0.28571429 -0.27142857 -0.25714286 -0.24285714 -0.22857143 -0.21428571 -0.2 -0.18571429 -0.17142857 -0.15714286 -0.14285714 -0.12857143 -0.11428571 -0.1 -0.08571429 -0.07142857 -0.05714286 -0.04285714 -0.02857143 -0.01428571 0 0 0 0 0 0
  line L47 (-136.2801, 44.0069) -> (-132.9329, 42.926)
  arc A95 (-131.6356, 40.4355) -> (-132.9329, 42.926) centre (-133.5475, 41.0228) ccw
  circle A96 centre (0, 0) radius 5
  circle A97 centre (264.6494, 4.9519) radius 5
  circle A98 centre (264.6494, 4.9519) radius 5
  dimension "d36" = 10
  constraint tangent A97 A98
  measures "d36" diameter of A97
sketch "Sketch2" plane through (0, 0, 0) normal (0, 0, 1) x (1, 0, 0)
sketch "Sketch3" plane through (0, 0, 10) normal (0, 0, 1) x (-1, 0, 0)
  circle A0 centre (0, 0) radius 5
  dimension "d37" = 10
  constraint coincident A0.centre origin
  measures "d37" diameter of A0
sketch "Sketch4" plane through (0, 0, 10) normal (0, 0, 1) x (-1, 0, 0)
  circle A0 centre (0, 0) radius 5
  dimension "d38" = 10
  constraint coincident A0.centre origin
  measures "d38" diameter of A0
extrude "Extrude3" add sketch "Sketch4" along normal blind 20 and the other way blind 32.17 sketch seen with x (0.991445, 0.130526, 0) y (-0.130526, 0.991445, 0) z (0, 0, 1) at (0, 0, 0) bodies 1 in component "Spur Gear 24 teeth"